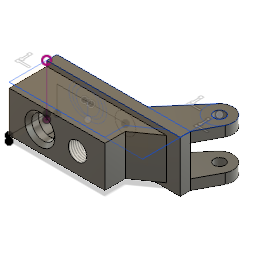
QWEwwe (2) (Autodesk Fusion 360 design; units mm, degrees)
Autodesk Fusion 360 part; units mm, degrees
sketch "Sketch1" plane through (0, 0, 0) normal (0, 1, 0) x (1, 0, 0)
  line L0 (-20, 15) -> (-20, -13)
  line L1 (-20, -13) -> (58, -13)
  line L2 (58, -13) -> (58, 15)
  line L3 (58, 15) -> (-20, 15)
  line L4 (58, -13) -> (58, 32)
  circle A0 centre (58, 32) radius 8
  line L5 (58, 15) -> (65.0588, 28.2353)
  line L6 (58, 15) -> (33, 15)
  line L7 (33, 15) -> (51.9113, 37.1892)
  circle A1 centre (58, 32) radius 3.3
  circle A2 centre (58, 32) radius 3.25
  line L8 (-20, -13) -> (36, -13)
  line L9 (58, 15) -> (58, 9)
  line L10 (58, 9) -> (50, 9)
  line L11 (36, -1) -> (50, 9)
  line L12 (36, -13) -> (36, -1)
  line L13 (58, 9) -> (-20, 9)
  dimension "d1" = 28
  dimension "d2" = 78
  dimension "d3" = 45
  dimension "d4" = 16
  dimension "d5" = 25
  dimension "d6" = 6.6
  dimension "d7" = 6.5
  dimension "d8" = 56
  dimension "d9" = 6
  dimension "d10" = 8
  measures "d3" distance of origin
  measures "d4" diameter of A0
  measures "d6" diameter of A1
  measures "d7" diameter of A2
extrude "Extrude1" add sketch "Sketch1" against normal blind 30 contours L0 L2 L3 L4 L6 L9 L10 L13 | L0 L1 L8 L11 L12 L13 | L3 L4 A0 L6 L7 | L1 L2 L4 L10 L11 L12 L13 | L4 A0 L5 | A0 | A1
extrude "Extrude2" cut sketch "Sketch1" against normal blind 3 contours L0 L1 L8 L11 L12 L13 | L1 L2 L4 L10 L11 L12 L13
extrude "Extrude3" cut sketch "Sketch1" against normal blind 53 contours L1 L2 L4 L10 L11 L12 L13
ref_plane "WorkPlane1" through (0, -6, 0) normal (0, 1, 0) x (0, 0, 1)
sketch "Sketch2" plane through (0, 0, 0) normal (0, 1, 0) x (1, 0, 0)
  line L0 (58, -13) -> (58, 32)
  line L1 (33, 15) -> (58, 15)
  circle A0 centre (58, 32) radius 8
  circle A1 centre (58, 32) radius 3.25
  line L2 (33, 15) -> (51.9113, 37.1892)
  line L3 (58, 15) -> (65.0588, 28.2353)
  line L4 (58, 15) -> (65.0588, 28.2353)
  line L5 (1, 0) -> (3, 0)
  line L6 (3, 0) -> (14, 0)
sketch "Sketch3" plane through (0, 0, -15) normal (0, 0, -1) x (-1, 0, 0)
  line L0 (20, 0) -> (-33, 0)
  line L1 (-33, 0) -> (-33, -30)
  line L2 (-33, -30) -> (20, -30)
  line L3 (20, -30) -> (20, 0)
  line L4 (20, -30) -> (20, -15)
  line L5 (20, -15) -> (2, -15)
  line L6 (2, -15) -> (2, -24)
  line L7 (2, -15) -> (0, -15)
  line L8 (2, -15) -> (4, -15)
  arc A0 (0, -6) -> (0, -24) centre (0, -15) ccw
  arc A1 (4, -24) -> (4, -6) centre (4, -15) ccw
  line L9 (4, -15) -> (4, -24) construction
  line L10 (4, -15) -> (4, -6) construction
  line L11 (4, -24) -> (0, -24)
  line L12 (4, -6) -> (0, -6)
  arc A2 (0, -8) -> (0, -22) centre (0, -15) ccw
  arc A3 (4, -22) -> (4, -8) centre (4, -15) ccw
  line L13 (4, -22) -> (0, -22)
  line L14 (4, -8) -> (0, -8)
  circle A4 centre (2, -15) radius 6.75
  line L15 (20, -15) -> (-20, -15)
  circle A5 centre (-20, -15) radius 6
  dimension "d18" = 2
  dimension "d19" = 9
  dimension "d20" = 180
  dimension "d21" = 13.5
  dimension "d30" = 40
  dimension "d31" = 12
  measures "d19" radius of A1
  measures "d20" angle of L9 L10
  measures "d21" diameter of A4
  measures "d31" diameter of A5
extrude "Extrude7" cut sketch "Sketch3" against normal blind 46 contours A5
extrude "Extrude4" cut sketch "Sketch3" against normal blind 48 contours L5 L6 L8 A4 L15 | L5 L7 L8 A4 L15 | L6 L7 A4 L15
extrude "Extrude5" cut sketch "Sketch3" against normal blind 22 contours L5 A2 A3 L14 A4 L15 | L5 L6 A3 L13 A4 L15 | L6 A2 L13 A4 L15
extrude "Extrude6" cut sketch "Sketch3" against normal blind 9 contours L5 A0 A1 L12 A2 A3 L14 L15 | L5 L6 A1 L11 A3 L13 L15 | L6 A0 L11 A2 L13 L15
chamfer "Chamfer1" distance 2 angle 45 4 edges at (-13, -15, -15) (-2, -24, -15) (9, -15, -15) (-2, -6, -15) measured on face at (-17.6583, -15.2242, -15) measured on face at (-17.6583, -15.2242, -15) measured on face at (-17.6583, -15.2242, -15) measured on face at (-17.6583, -15.2242, -15)
thread "Thread1" "ISO Metric profile 12.0 M12x1.25 6H" major diameter 12.18 minor diameter 10.7795 pitch 1.25 angle 60 resizes the face on face at (14.0298, -15.5974, 3.6667)
sketch "Sketch4" plane through (-20, 0, 0) normal (-1, 0, 0) x (0, 0, 1)
  line L0 (-9, -3) -> (-9, 0)
  line L1 (-9, 0) -> (-15, 0)
  line L2 (-15, 0) -> (-15, -30)
  line L3 (-15, -30) -> (13, -30)
  line L4 (13, -30) -> (13, -3)
  line L5 (13, -3) -> (-9, -3)
  line L6 (13, -30) -> (13, -27)
  line L7 (-9, 0) -> (-9, -30)
  line L8 (13, -27) -> (-9, -27)
  line L9 (-9, -27) -> (-9, -30)
  dimension "d34" = 3
extrude "Extrude8" cut sketch "Sketch4" against normal blind 104 contours L3 L4 L6 L7 L8 L9
extrude "Extrude9" cut sketch "Sketch2" sketch "Sketch1" against normal blind 24 contours L0 L1 A0 L2 | A0 of sketch 2 contours L4 A0 L5 | A0 | A1
extrude "Extrude10" add sketch "Sketch1" against normal blind 6 contours L3 L4 A0 L6 L7 | L4 A0 L5 | A0 | A1
chamfer "Chamfer2" distance 2 angle 45 1 edges at (4.2932, -17.4409, 13) measured on face at (-16.25, -15, 13)
